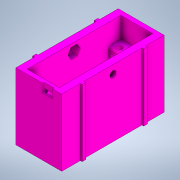
# Autodesk Inventor part: hull_servo
Saved by Autodesk Inventor 2020 (Build 240168000, 168)
## iProperties
Created: 2019-09-18
Part Number: hull_servo
Material: Generic
Document SubType Name: Modeling
Designer: suchanek
Density: 1 g/cm^3
Appearance: Default
Author: suchanek
Autodesk Inventor part; units mm, degrees
ref_plane "YZ Plane" through (0, 0, 0) normal (1, 0, 0) x (0, 1, 0)
ref_plane "XZ Plane" through (0, 0, 0) normal (0, 1, 0) x (-1, 0, 0)
ref_plane "XY Plane" through (0, 0, 0) normal (0, 0, 1) x (1, 0, 0)
sketch "Sketch1" plane through (0, 0, 0) normal (0, 1, 0) x (-1, 0, 0)
  line L0 (-15.5, 33.5) -> (15.5, 33.5)
  line L1 (15.5, 33.5) -> (15.5, -33.5)
  line L2 (15.5, -33.5) -> (-15.5, -33.5)
  line L3 (-15.5, -33.5) -> (-15.5, 33.5)
  line L4 (-15.5, 33.5) -> (15.5, -33.5) construction
  line L5 (15.5, 33.5) -> (-15.5, -33.5) construction
  line L6 (-22.3, 49.8) -> (22.3, 49.8)
  line L7 (22.3, 49.8) -> (22.3, -49.8)
  line L8 (22.3, -49.8) -> (-22.3, -49.8)
  line L9 (-22.3, -49.8) -> (-22.3, 49.8)
  line L10 (-22.3, 49.8) -> (22.3, -49.8) construction
  line L11 (22.3, 49.8) -> (-22.3, -49.8) construction
  line L12 (22.3, -28.2) -> (24.1, -28.2)
  line L13 (24.1, -28.2) -> (24.1, -31.8)
  line L14 (24.1, -31.8) -> (22.3, -31.8)
  line L15 (22.3, -31.8) -> (22.3, -28.2)
  line L16 (0, 0) -> (0, -11.0909)
  line L17 (0, -11.0909) -> (0, 0)
  line L18 (0, 0) -> (9.2257, 0)
  line L19 (22.3, 28.2) -> (24.1, 28.2)
  line L20 (24.1, 28.2) -> (24.1, 31.8)
  line L21 (24.1, 31.8) -> (22.3, 31.8)
  line L22 (22.3, 31.8) -> (22.3, 28.2)
  line L23 (-22.3, -28.2) -> (-24.1, -28.2)
  line L24 (-24.1, -28.2) -> (-24.1, -31.8)
  line L25 (-24.1, -31.8) -> (-22.3, -31.8)
  line L26 (-22.3, -31.8) -> (-22.3, -28.2)
  line L27 (-22.3, 28.2) -> (-24.1, 28.2)
  line L28 (-22.3, 31.8) -> (-22.3, 28.2)
  line L29 (-24.1, 31.8) -> (-22.3, 31.8)
  line L30 (-24.1, 28.2) -> (-24.1, 31.8)
  point P0 (22.3, -31.8)
  point P1 (-22.3, -31.8)
  point P2 (-22.3, -28.2)
  point P3 (-22.3, 28.2)
  point P4 (-22.3, 31.8)
  point P5 (22.3, 31.8)
  dimension "d0" = 31
  dimension "d1" = 67
  dimension "d2" = 44.6
  dimension "d3" = 99.6
  dimension "d11" = 1.8
  dimension "d12" = 3.6
  dimension "d13" = 28.2
  constraints: 62 end point, 12 symmetric about line, 7 equal length, 4 horizontal, 4 midpoint, 3 perpendicular, 1 point on line, 1 vertical
  measures "d0" distance of L1.end L2.end
  measures "d1" distance of L0.end L1.end
  measures "d2" distance of L7.end L8.end
  measures "d3" distance of L6.end L7.end
  measures "d11" distance of L13.end L14.end
  measures "d12" distance of L12.end L13.end
  measures "d13" distance from line of L16.start L12
extrude "Extrusion1" add sketch "Sketch1" against normal blind 7 contours L0 L1 L2 L3 | L6 L7 L8 L9 | L9 L27 L30 L29 | L21 L20 L19 L7 | L9 L25 L24 L23 | L12 L13 L14 L7
extrude "Extrusion2" add sketch "Sketch1" along normal blind 58
sketch "Sketch2" plane through (0, 58, 0) normal (0, 1, 0) x (1, 0, 0)
  line L0 (-15.5, -45.5) -> (15.5, -45.5)
  line L1 (15.5, -45.5) -> (15.5, 45.5)
  line L2 (15.5, 45.5) -> (-15.5, 45.5)
  line L3 (-15.5, 45.5) -> (-15.5, -45.5)
  line L4 (-15.5, -45.5) -> (15.5, 45.5) construction
  line L5 (15.5, -45.5) -> (-15.5, 45.5) construction
  line L6 (-15.5, 33.5) -> (-15.5, -33.5) projected
  line L7 (-15.5, -33.5) -> (15.5, -33.5) projected
  line L8 (15.5, -33.5) -> (15.5, 33.5) projected
  line L9 (15.5, 33.5) -> (-15.5, 33.5) projected
  point P0 (0, 0)
  point P1 (15.5, 33.5)
  point P2 (15.5, -33.5)
  dimension "d8" = 12
  constraints: 12 end point, 2 midpoint, 2 parallel, 1 collinear, 1 horizontal, 1 perpendicular
  measures "d8" distance between parallel lines of L0 L7
extrude "Extrusion3" cut sketch "Sketch2" against normal blind 20 contours L3 L7 L1 L0 | L3 L2 L1 L9
sketch "Sketch3" plane through (22.3, -7, 28.2) normal (1, 0, 0) x (0, 0, -1)
  line L0 (0, 0) -> (0, 65) projected
  line L1 (0, 65) -> (56.4, 65) projected
  line L2 (56.4, 0) -> (56.4, 65) projected
  circle A0 centre (28.2, 57) radius 3
  point P0 (28.2, 7)
  dimension "d18" = 6
  dimension "d19" = 8
  constraints: 1 centre point, 1 vertical alignment
  measures "d18" diameter of A0
  measures "d19" distance from line of L1 A0.centre
extrude "Extrusion4" cut sketch "Sketch3" against normal through all
sketch "Sketch6" plane through (15.5, 0, 33.5) normal (0, 0, -1) x (-1, 0, 0)
  line L0 (31, 0) -> (0, 0) projected
  line L1 (31, 38) -> (0, 38) projected
  line L2 (12, 0) -> (19, 0)
  line L3 (19, 0) -> (19, 38)
  line L4 (19, 38) -> (12, 38)
  line L5 (12, 38) -> (12, 0)
  line L6 (15.5, 0) -> (15.5, 3.571)
  dimension "d23" = 7
  constraints: 10 end point, 2 parallel, 2 point on line, 1 horizontal, 1 perpendicular, 1 vertical, 1 other
  measures "d23" distance between parallel lines of L3 L5
extrude "Extrusion6" cut sketch "Sketch6" against normal blind 4
sketch "Sketch7" plane through (0, 38, 0) normal (0, 1, 0) x (1, 0, 0)
  line L0 (3.5, -37.5) -> (-3.5, -37.5) projected
  line L1 (15.5, -45.5) -> (-15.5, -45.5) projected
  line L2 (-3.5, -37.5) -> (3.5, -37.5)
  line L3 (3.5, -37.5) -> (3.5, -45.5)
  line L4 (3.5, -45.5) -> (-3.5, -45.5)
  line L5 (-3.5, -45.5) -> (-3.5, -37.5)
  line L6 (3.5, -33.5) -> (3.5, -37.5) projected
  point P0 (0, 0)
  constraints: 8 end point, 2 parallel, 1 collinear, 1 horizontal, 1 perpendicular, 1 point on line
extrude "Extrusion7" cut sketch "Sketch7" against normal blind 5
sketch "Sketch8" plane through (15.5, 58, 45.5) normal (0, 0, -1) x (-1, 0, 0)
  line L0 (19, -20) -> (19, -25) projected
  line L1 (19, -25) -> (12, -25)
  line L2 (12, -25) -> (3.7, -8)
  line L3 (3.7, -8) -> (10.7, -8)
  line L4 (10.7, -8) -> (19, -25)
  line L5 (12, -58) -> (12, -20) projected
  line L6 (12.2, -8) -> (2.2, -8)
  line L7 (2.2, -8) -> (2.2, -5)
  line L8 (2.2, -5) -> (12.2, -5)
  line L9 (12.2, -5) -> (12.2, -8)
  line L10 (15.5, -25) -> (15.5, -21)
  line L11 (0, 0) -> (31, 0) projected
  line L12 (7.2, -8) -> (7.2, -9.1471)
  point P0 (15.5, -58)
  point P1 (16.5, -20)
  point P2 (-6.8, 0)
  dimension "d28" = 3
  dimension "d29" = 10
  dimension "d30" = 5
  dimension "d36" = 9
  constraints: 20 end point, 4 parallel, 2 horizontal, 2 midpoint, 2 vertical, 1 collinear, 1 perpendicular, 1 point on line, 1 symmetric about line, 1 other
  measures "d28" distance of L8.end L6.start
  measures "d29" distance of L7.end L8.end
  measures "d30" distance between parallel lines of L11 L8
  measures "d36" distance from line of point (-6.8, 0) L7
extrude "Extrusion8" cut sketch "Sketch8" against normal blind 3 contours L1 L2 L3 L4
extrude "Extrusion9" cut sketch "Sketch8" against normal through all contours L3 L6 L7 L8 L9
fillet "Fillet1" radius 7 1 edges at (0, 33, 37.5)
fillet "Fillet2" radius 3 2 edges at (9.5, 38, 33.5) (-9.5, 38, 33.5)
fillet "Fillet4" radius 3 1 edges at (0, 38, -33.5)
sketch "Sketch10" plane through (-15.5, 0, 33.5) normal (1, 0, 0) x (0, 0, -1)
  circle A0 centre (33.5, 50) radius 3 projected
  line L0 (36.5022, 55.2) -> (39.5044, 50)
  line L1 (39.5044, 50) -> (36.5022, 44.8)
  line L2 (36.5022, 44.8) -> (30.4978, 44.8)
  line L3 (30.4978, 44.8) -> (27.4956, 50)
  line L4 (27.4956, 50) -> (30.4978, 55.2)
  line L5 (30.4978, 55.2) -> (36.5022, 55.2)
  line L6 (-12, 58) -> (79, 58) projected
  point P0 (33.5, 0)
  dimension "d45" = 10.4
  constraints: 12 end point, 1 coincident, 1 parallel, 13 other
  measures "d45" distance between parallel lines of L2 L5
extrude "Extrusion11" cut sketch "Sketch10" along normal blind 35.8 and the other way blind 4.8
sketch "Sketch11" plane through (0, 58, 0) normal (0, 1, 0) x (1, 0, 0)
  circle A0 centre (-8.8, -37.5) radius 2.75
  line L0 (0, 0) -> (-3.9121, 0)
  line L1 (0, 0) -> (0, -5.8643)
  circle A1 centre (8.8, -37.5) radius 2.75
  circle A2 centre (-8.8, 37.5) radius 2.75
  circle A3 centre (8.8, 37.5) radius 2.75
  dimension "d50" = 5.5
  dimension "d51" = 17.6
  dimension "d52" = 75
  constraints: 4 centre point, 4 end point, 3 symmetric about line, 1 horizontal, 1 vertical, 3 other
  measures "d50" diameter of A0
  measures "d51" distance of A1.centre A0.centre
  measures "d52" distance of A2.centre A0.centre
extrude "Extrusion12" cut sketch "Sketch11" against normal blind 50
ref_plane "Work Plane1" through (0, 28, 0) normal (0, 1, 0) x (1, 0, 0)
sketch "Sketch12" plane through (0, 28, 0) normal (0, 1, 0) x (1, 0, 0)
  line L0 (-6.3463, -33.25) -> (-3.8925, -37.5)
  line L1 (-3.8925, -37.5) -> (-6.3463, -41.75)
  line L2 (-6.3463, -41.75) -> (-11.2537, -41.75)
  line L3 (-11.2537, -41.75) -> (-13.7075, -37.5)
  line L4 (-13.7075, -37.5) -> (-11.2537, -33.25)
  line L5 (-11.2537, -33.25) -> (-6.3463, -33.25)
  circle A0 centre (-8.8, -37.5) radius 2.75 projected
  line L6 (-13.7075, -37.5) -> (-3.8925, -37.5)
  line L7 (-3.8925, -37.5) -> (-3.8925, -33.25)
  line L8 (-3.8925, -33.25) -> (-13.7075, -33.25)
  line L9 (-13.7075, -33.25) -> (-13.7075, -37.5)
  line L10 (0, 0) -> (-6.05, 0)
  line L11 (0, 0) -> (0, -8.2148)
  line L12 (6.3463, -33.25) -> (3.8925, -37.5)
  line L13 (3.8925, -37.5) -> (6.3463, -41.75)
  line L14 (6.3463, -41.75) -> (11.2537, -41.75)
  line L15 (11.2537, -41.75) -> (13.7075, -37.5)
  line L16 (13.7075, -37.5) -> (11.2537, -33.25)
  line L17 (11.2537, -33.25) -> (6.3463, -33.25)
  circle A1 centre (8.8, -37.5) radius 2.75
  line L18 (13.7075, -37.5) -> (3.8925, -37.5)
  line L19 (3.8925, -37.5) -> (3.8925, -33.25)
  line L20 (3.8925, -33.25) -> (13.7075, -33.25)
  line L21 (13.7075, -33.25) -> (13.7075, -37.5)
  line L22 (-6.3463, 33.25) -> (-3.8925, 37.5)
  line L23 (-3.8925, 37.5) -> (-6.3463, 41.75)
  line L24 (-6.3463, 41.75) -> (-11.2537, 41.75)
  line L25 (-11.2537, 41.75) -> (-13.7075, 37.5)
  line L26 (-13.7075, 37.5) -> (-11.2537, 33.25)
  line L27 (-11.2537, 33.25) -> (-6.3463, 33.25)
  circle A2 centre (-8.8, 37.5) radius 2.75
  line L28 (-13.7075, 37.5) -> (-3.8925, 37.5)
  line L29 (-3.8925, 37.5) -> (-3.8925, 33.25)
  line L30 (-3.8925, 33.25) -> (-13.7075, 33.25)
  line L31 (-13.7075, 33.25) -> (-13.7075, 37.5)
  line L32 (6.3463, 33.25) -> (3.8925, 37.5)
  line L33 (3.8925, 37.5) -> (6.3463, 41.75)
  line L34 (6.3463, 41.75) -> (11.2537, 41.75)
  line L35 (11.2537, 41.75) -> (13.7075, 37.5)
  line L36 (13.7075, 37.5) -> (11.2537, 33.25)
  line L37 (11.2537, 33.25) -> (6.3463, 33.25)
  circle A3 centre (8.8, 37.5) radius 2.75
  line L38 (13.7075, 37.5) -> (3.8925, 37.5)
  line L39 (3.8925, 37.5) -> (3.8925, 33.25)
  line L40 (3.8925, 33.25) -> (13.7075, 33.25)
  line L41 (13.7075, 33.25) -> (13.7075, 37.5)
  dimension "d56" = 8.5
  constraints: 84 end point, 33 symmetric about line, 4 coincident, 4 point on line, 3 centre point, 3 horizontal, 2 parallel, 1 collinear, 1 perpendicular, 1 vertical, 16 other
  measures "d56" distance between parallel lines of L3 L0
extrude "Extrusion13" cut sketch "Sketch12" along normal blind 4.5
sketch "Sketch13" plane through (0, 0, 0) normal (0, 1, 0) x (1, 0, 0)
  line L0 (3.5, -33.5) -> (3.5, -37.5) projected
  line L1 (-15.5, 33.5) -> (15.5, 33.5) projected
  line L2 (3.5, -37.5) -> (-3.5, -37.5)
  line L3 (-3.5, -37.5) -> (-3.5, 33.5)
  line L4 (-3.5, 33.5) -> (3.5, 33.5)
  line L5 (3.5, 33.5) -> (3.5, -37.5)
  line L6 (-3.5, -45.5) -> (-3.5, -36.5) projected
  point P0 (0, 0)
  constraints: 8 end point, 2 parallel, 1 collinear, 1 horizontal, 1 perpendicular, 1 point on line
extrude "Extrusion14" cut sketch "Sketch13" against normal blind 2
sketch "Sketch14" plane through (-15.5, 0, -33.5) normal (0, 0, 1) x (1, 0, 0)
  line L0 (12, -2) -> (19, -2) projected
  line L1 (19, -2) -> (12, -2)
  line L2 (12, -2) -> (12, 38)
  line L3 (12, 38) -> (19, 38)
  line L4 (19, 38) -> (19, -2)
  line L5 (12, 0) -> (12, -2) projected
  line L6 (21.7383, 38) -> (9.2617, 38) projected
  point P0 (15.5, 0)
  constraints: 8 end point, 2 collinear, 2 parallel, 1 horizontal, 1 perpendicular
extrude "Extrusion15" cut sketch "Sketch14" against normal blind 7
draft "FaceDraft1" angle -3 pull direction (0, 1, 0) faces at (1.1667, 11.3333, -40.5) fixed edges at (0, -2, -40.5)
sketch "Sketch15" plane through (-22.3, -7, 49.8) normal (0, 0, 1) x (1, 0, 0)
  line L0 (35.6, 60) -> (25.6, 60) projected
  line L1 (25.6, 60) -> (35.6, 60)
  line L2 (35.6, 60) -> (35.6, 65)
  line L3 (35.6, 65) -> (25.6, 65)
  line L4 (25.6, 65) -> (25.6, 60)
  line L5 (35.6, 60) -> (35.6, 57) projected
  line L6 (0, 65) -> (44.6, 65) projected
  point P0 (22.3, 7)
  constraints: 8 end point, 2 collinear, 2 parallel, 1 horizontal, 1 perpendicular
extrude "Extrusion16" cut sketch "Sketch15" against normal blind 1.5
body "Solid1"
